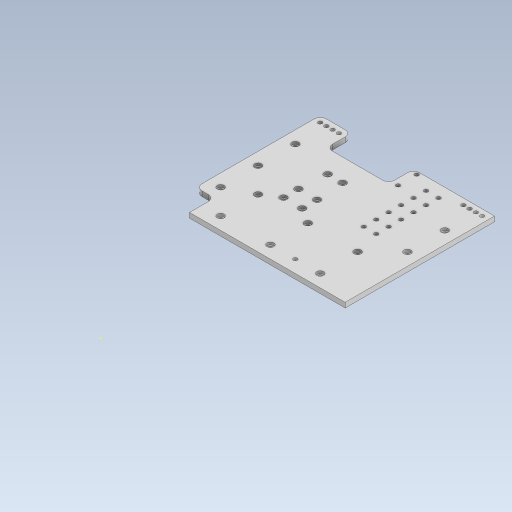
# Autodesk Inventor part: Fix Casis Kanan Bawah
Saved by Autodesk Inventor 2023.5 (Build 275446000, 446)
## iProperties
Created: 2025-10-01
Part Number: Fix Casis Kanan Bawah
Material: Generic
Document SubType Name: Modeling
Designer: Guntur
Density: 1 g/cm^3
Appearance: Default
Author: Guntur
## iProperties of the stored document Fix Casis Kanan Depan_3DPrint.ipt
Created: 2025-10-18
Part Number: Fix Casis Kanan Depan_3DPrint
Material: Generic
Document SubType Name: Modeling
Designer: Guntur
Density: 1 g/cm^3
Appearance: Default
Author: Guntur
Autodesk Inventor part; units mm, degrees
ref_plane "YZ Plane" through (0, 0, 0) normal (1, 0, 0) x (0, 1, 0)
ref_plane "XZ Plane" through (0, 0, 0) normal (0, 1, 0) x (-1, 0, 0)
ref_plane "XY Plane" through (0, 0, 0) normal (0, 0, 1) x (1, 0, 0)
sketch "Sketch1" plane through (0, 0, 0) normal (0, 1, 0) x (-1, 0, 0)
  circle A0 centre (51.9082, -238.2442) radius 1.6
  circle A1 centre (46.9082, -238.2442) radius 1.6
  line L0 (41.8423, -223.2442) -> (41.8423, -243.2442)
  line L1 (41.8423, -243.2442) -> (-8.0918, -243.2442)
  line L2 (-8.0918, -223.2442) -> (41.8423, -223.2442)
  line L3 (-8.0918, -243.2442) -> (-8.0918, -223.2442)
  circle A2 centre (56.9082, -238.2442) radius 1.6
  circle A3 centre (61.9082, -238.2442) radius 1.6
  circle A4 centre (9.4082, -171.2442) radius 2.75
  line L4 (66.8423, -243.2442) -> (-73.1577, -243.2442)
  line L5 (66.8423, -123.2442) -> (66.8423, -243.2442)
  line L6 (-3.1577, -123.2442) -> (-3.1577, -243.2442) construction
  line L7 (71.8423, -183.2442) -> (-68.1577, -183.2442) construction
  line L8 (-73.1577, -123.2442) -> (66.8423, -123.2442)
  line L9 (-73.1577, -243.2442) -> (-73.1577, -123.2442)
  circle A5 centre (-63.1577, -213.2442) radius 1.6
  circle A6 centre (-63.1577, -183.2442) radius 1.6
  circle A7 centre (-63.1577, -183.2442) radius 2.75
  circle A8 centre (-63.1577, -213.2442) radius 2.75
  circle A9 centre (-68.0918, -238.2442) radius 1.6
  circle A10 centre (-63.0918, -238.2442) radius 1.6
  circle A11 centre (-58.0918, -238.2442) radius 1.6
  circle A12 centre (-53.0918, -238.2442) radius 1.6
  circle A13 centre (9.4082, -171.2442) radius 1.6
  circle A14 centre (24.4082, -171.2442) radius 1.6
  circle A15 centre (24.4082, -171.2442) radius 2.75
  circle A16 centre (9.4082, -183.2442) radius 1.6
  circle A17 centre (9.4082, -183.2442) radius 2.75
  circle A18 centre (24.4082, -183.2442) radius 1.6
  circle A19 centre (24.4082, -183.2442) radius 2.75
  circle A20 centre (10.9082, -205.2442) radius 1.6
  circle A21 centre (10.9082, -205.2442) radius 2.75
  circle A22 centre (22.9082, -205.2442) radius 1.6
  circle A23 centre (22.9082, -205.2442) radius 2.75
  circle A24 centre (-43.1577, -133.2442) radius 1.6
  circle A25 centre (-43.1577, -133.2442) radius 2.75
  circle A26 centre (-3.1577, -133.2442) radius 1.6
  circle A27 centre (-3.1577, -133.2442) radius 2.75
  circle A28 centre (36.8423, -133.2442) radius 1.6
  circle A29 centre (36.8423, -133.2442) radius 2.75
  circle A30 centre (56.9082, -128.2442) radius 1.6
  circle A31 centre (61.9082, -128.2442) radius 1.6
  circle A32 centre (56.8423, -213.2442) radius 1.6
  circle A33 centre (56.8423, -213.2442) radius 2.75
  circle A34 centre (56.8423, -183.2442) radius 1.6
  circle A35 centre (56.8423, -183.2442) radius 2.75
  circle A36 centre (56.8423, -153.2442) radius 1.6
  circle A37 centre (56.8423, -153.2442) radius 2.75
  circle A38 centre (-13.0918, -240.7442) radius 1.6
  circle A39 centre (-13.0918, -225.7442) radius 1.6
  circle A40 centre (-38.0918, -233.2442) radius 1.6
  circle A41 centre (-28.0918, -233.2442) radius 1.6
  circle A42 centre (-28.0918, -223.2442) radius 1.6
  circle A43 centre (-38.0918, -223.2442) radius 1.6
  circle A44 centre (-28.0918, -203.2442) radius 1.6
  circle A45 centre (-28.0918, -213.2442) radius 1.6
  circle A46 centre (-38.0918, -203.2442) radius 1.6
  circle A47 centre (-38.0918, -213.2442) radius 1.6
  line L10 (-33.0918, -198.2442) -> (-28.0918, -198.2442)
  circle A48 centre (-28.0918, -183.2442) radius 1.6
  circle A49 centre (-38.0918, -183.2442) radius 1.6
  circle A50 centre (-38.0918, -193.2442) radius 1.6
  circle A51 centre (-28.0918, -193.2442) radius 1.6
  circle A52 centre (36.8423, -163.2442) radius 1.65
  circle A53 centre (36.8423, -163.2442) radius 2.75
  circle A54 centre (-3.1577, -163.2442) radius 1.65
  circle A55 centre (-3.1577, -163.2442) radius 2.75
  circle A56 centre (-43.1577, -163.2442) radius 1.65
  circle A57 centre (-43.1577, -163.2442) radius 2.75
  line L11 (66.8423, -123.2442) -> (51.8423, -123.2442)
  line L12 (51.8423, -123.2442) -> (51.8423, -143.2442)
  line L13 (51.8423, -143.2442) -> (66.8423, -143.2442)
  line L14 (66.8423, -143.2442) -> (66.8423, -123.2442)
  circle A58 centre (-23.1577, -133.2442) radius 1.6
  point P0 (0, -190.5)
  point P1 (16.9082, -168.6317)
  point P2 (16.9082, -205.2442)
  dimension "d33" = 140
  dimension "d34" = 120
  dimension "d35" = 10
  dimension "d36" = 10
  dimension "d37" = 10
  dimension "d39" = 10
  dimension "d40" = 10
  dimension "d41" = 10
  dimension "d42" = 10
  dimension "d43" = 10
  dimension "d44" = 40
  dimension "d45" = 40
  dimension "d46" = 3.2
  dimension "d47" = 2.5
  dimension "d48" = 5
  dimension "d49" = 3.2
  dimension "d50" = 15
  dimension "d60" = 3.2
  dimension "d61" = 3.2
  dimension "d63" = 3.2
  dimension "d65" = 3.2
  dimension "d66" = 10
  dimension "d69" = 10
  dimension "d70" = 10
  dimension "d71" = 10
  dimension "d76" = 3.3
  dimension "d77" = 5.5
  dimension "d78" = 30
  dimension "d79" = 3.3
  dimension "d80" = 5.5
  dimension "d81" = 15
  dimension "d82" = 20
  dimension "d84" = 3.2
  dimension "d85" = 20
  constraints: 59 centre point, 26 end point, 17 coincident, 6 symmetric about line, 5 point on line, 2 parallel, 1 horizontal, 1 perpendicular, 12 other
  measures "d33" distance of L4.start L4.end
  measures "d34" distance of L4.end L8.start
  measures "d35" distance from line of L8 A29.centre
  measures "d36" distance from line of L8 A27.centre
  measures "d37" distance from line of L8 A25.centre
  measures "d44" distance from line of A25.centre L6
  measures "d45" distance from line of L6 A28.centre
  measures "d46" diameter of A38
  measures "d47" distance from line of L4 A38.centre
  measures "d48" distance from line of L3 A38.centre
  measures "d49" diameter of A39
  measures "d50" distance of A38.centre A39.centre
  measures "d60" diameter of A43
  measures "d61" diameter of A40
  measures "d63" diameter of A41
  measures "d65" diameter of A42
  measures "d66" distance of A43.centre A42.centre
  measures "d69" distance from line of L4 A40.centre
  measures "d70" distance of A40.centre A43.centre
  measures "d71" distance from line of L4 A41.centre
  measures "d76" diameter of A52
  measures "d77" diameter of A53
  measures "d78" distance of A52.centre A29.centre
  measures "d79" diameter of A54
  measures "d80" diameter of A55
  measures "d81" distance of L13.end L12.end
  measures "d82" distance of L12.end L11.end
  measures "d84" diameter of A58
  measures "d85" distance of A58.centre A25.centre
extrude "Extrusion1" add sketch "Sketch1" along normal blind 4 contours L2 L3 L4 L9 L8 L12 L13 L5 L0
sketch "Sketch2" plane through (0, 4, 0) normal (0, 1, 0) x (1, 0, 0)
  point P0 (0, 0)
extrude "Extrusion2" add sketch "Sketch1" along normal blind 2 contours L2 L3 L4 L9 L8 L12 L13 L5 L0 | A4 | A7 | A8 | A15 | A17 | A19 | A21 | A23 | A25 | A27 | A29 | A33 | A35 | A37 | A53 | A55 | A57
fillet "Fillet1" radius 5 7 edges at (-51.8423, 2, -143.2442) (-66.8423, 2, -143.2442) (-66.8423, 2, -243.2442) (8.0918, 2, -243.2442) (8.0918, 2, -223.2442) (-41.8423, 2, -223.2442) (-41.8423, 2, -243.2442)
body "Solid1"
